376830ed-f0d3-40e7-8504-639e06eeb14b (Autodesk Fusion 360 design; units mm, degrees)
Autodesk Fusion 360 part; units mm, degrees
note: some values were not read from the file. Set by a fixed rule: which sketch regions a step uses.
sketch "Sketch1" plane through (0, 0, 0) normal (0, 1, 0) x (1, 0, 0)
  circle A0 centre (0, 0) radius 8.4709
  circle A1 centre (0, 0) radius 9.525
  circle A2 centre (0, 0) radius 7.412
  circle A3 centre (0, 0) radius 7.96
  arc A4 (9.5006, -0.6814) -> (-8.7304, -3.8087) centre (0, 0) ccw
  circle A5 centre (0, 0) radius 2.3813
  line L0 (0, 0) -> (9.525, 0) construction
  line L1 (0, 0) -> (-0.6938, -7.9298)
  line L2 (0, 0) -> (-1.3822, -7.8391)
  line L3 (0, 0) -> (-2.0602, -7.6888)
  line L4 (0, 0) -> (-2.7225, -7.48)
  line L5 (0, 0) -> (-3.3641, -7.2142)
  line L6 (0, 0) -> (-3.98, -6.8936)
  line L7 (0, 0) -> (-4.5657, -6.5205)
  line L8 (-0.6938, -7.9298) -> (-0.0018, -7.9903) construction
  line L9 (-1.3822, -7.8391) -> (-0.0141, -8.0804) construction
  line L10 (-2.0602, -7.6888) -> (-0.0473, -8.2282) construction
  line L11 (-2.7225, -7.48) -> (-0.1115, -8.4303) construction
  line L12 (-3.3641, -7.2142) -> (-0.2162, -8.6821) construction
  line L13 (-3.98, -6.8936) -> (-0.3705, -8.9775) construction
  line L14 (-4.5657, -6.5205) -> (-0.5826, -9.3095) construction
  line L15 (0, 0) -> (-5.1166, -6.0977)
  line L16 (-5.1166, -6.0977) -> (-0.8596, -9.6698) construction
  line L17 (0, 0) -> (-5.6286, -5.6286)
  line L18 (-5.6286, -5.6286) -> (-1.2079, -10.0493) construction
  spline S0 degree 5 poles (-1.2079, -10.0493) (-1.1965, -10.0361) (-1.1735, -10.01) (-1.139, -9.9713) (-1.0926, -9.9208) (-1.0346, -9.8592) (-0.9772, -9.7985) (-0.9208, -9.7382) (-0.8662, -9.678) (-0.8137, -9.6174) (-0.7634, -9.5563) (-0.7154, -9.4949) (-0.6695, -9.4332) (-0.6254, -9.3717) (-0.5829, -9.3104) (-0.5419, -9.2498) (-0.5022, -9.1898) (-0.4639, -9.1306) (-0.4271, -9.072) (-0.3918, -9.0141) (-0.3582, -8.9569) (-0.3264, -8.9002) (-0.2962, -8.8442) (-0.2677, -8.789) (-0.2409, -8.7347) (-0.2156, -8.6813) (-0.1919, -8.629) (-0.1697, -8.5779) (-0.1489, -8.5281) (-0.1297, -8.4795) (-0.112, -8.4323) (-0.0958, -8.3866) (-0.081, -8.3424) (-0.0676, -8.2999) (-0.0557, -8.2592) (-0.045, -8.2203) (-0.0356, -8.1835) (-0.0275, -8.1488) (-0.0206, -8.1164) (-0.015, -8.0864) (-0.0104, -8.059) (-0.0068, -8.0343) (-0.0041, -8.0127) (-0.0021, -7.9944) (-0.0007, -7.9796) (0.0002, -7.9687) (0.0004, -7.9631) (0.0003, -7.9609) (0.0001, -7.9602) (0, -7.96) knots 0 0 0 0 0 0 0.022222 0.044444 0.066667 0.088889 0.111111 0.133333 0.155556 0.177778 0.2 0.222222 0.244444 0.266667 0.288889 0.311111 0.333333 0.355556 0.377778 0.4 0.422222 0.444444 0.466667 0.488889 0.511111 0.533333 0.555556 0.577778 0.6 0.622222 0.644444 0.666667 0.688889 0.711111 0.733333 0.755556 0.777778 0.8 0.822222 0.844444 0.866667 0.888889 0.911111 0.933333 0.955556 0.977778 1 1 1 1 1 1
  line L19 (-1.3092, -10.166) -> (-1.1066, -9.9326)
  line L20 (0.0095, -7.9702) -> (-0.0095, -7.9499)
  line L21 (-0.1263, -8.47) -> (0, 0)
  line L22 (0, 0) -> (-0.6891, -6.0674) construction
  line L23 (0, -7.96) -> (0, 0) construction
  spline S1 degree 5 poles (0, -7.96) (0, -7.9287) (0, -7.8696) (0, -7.7913) (0, -7.7043) (0, -7.6106) (0, -7.5366) (0, -7.4767) (0, -7.434) (0, -7.412) knots 0 0 0 0 0 0 0.2 0.4 0.6 0.8 1 1 1 1 1 1
  spline S2 degree 5 poles (-1.785, -7.7573) (-1.7779, -7.7268) (-1.7647, -7.6691) (-1.7471, -7.5928) (-1.7276, -7.5081) (-1.7066, -7.4168) (-1.69, -7.3446) (-1.6766, -7.2863) (-1.667, -7.2447) (-1.6621, -7.2233) knots 0 0 0 0 0 0 0.2 0.4 0.6 0.8 1 1 1 1 1 1
  line L24 (0, -8.0339) -> (0, -7.8862)
  line L25 (0, -7.4639) -> (0, -7.3602)
  line L26 (-1.8015, -7.8293) -> (-1.7684, -7.6854)
  line L27 (-1.6737, -7.2738) -> (-1.6505, -7.1728)
  spline S3 degree 5 poles (-1.0763, -10.0642) (-1.0845, -10.0488) (-1.101, -10.0182) (-1.126, -9.9728) (-1.1599, -9.9132) (-1.2025, -9.8401) (-1.2449, -9.7681) (-1.2863, -9.6967) (-1.3261, -9.6258) (-1.3637, -9.5549) (-1.399, -9.4841) (-1.432, -9.4135) (-1.4629, -9.3431) (-1.492, -9.2732) (-1.5197, -9.2041) (-1.5461, -9.1358) (-1.5713, -9.0684) (-1.5953, -9.0021) (-1.6181, -8.9368) (-1.6395, -8.8725) (-1.6594, -8.8091) (-1.6778, -8.7467) (-1.6946, -8.6854) (-1.71, -8.6252) (-1.7239, -8.5662) (-1.7366, -8.5086) (-1.748, -8.4523) (-1.7582, -8.3975) (-1.7672, -8.3443) (-1.7751, -8.2927) (-1.7818, -8.2427) (-1.7873, -8.1945) (-1.7918, -8.1481) (-1.7953, -8.1037) (-1.7978, -8.0613) (-1.7995, -8.0211) (-1.8004, -7.9831) (-1.8005, -7.9475) (-1.7999, -7.9143) (-1.7987, -7.8838) (-1.797, -7.8561) (-1.795, -7.8312) (-1.7928, -7.8096) (-1.7906, -7.7913) (-1.7887, -7.7766) (-1.7871, -7.7657) (-1.786, -7.7602) (-1.7854, -7.758) (-1.7851, -7.7574) (-1.785, -7.7573) knots 0 0 0 0 0 0 0.022222 0.044444 0.066667 0.088889 0.111111 0.133333 0.155556 0.177778 0.2 0.222222 0.244444 0.266667 0.288889 0.311111 0.333333 0.355556 0.377778 0.4 0.422222 0.444444 0.466667 0.488889 0.511111 0.533333 0.555556 0.577778 0.6 0.622222 0.644444 0.666667 0.688889 0.711111 0.733333 0.755556 0.777778 0.8 0.822222 0.844444 0.866667 0.888889 0.911111 0.933333 0.955556 0.977778 1 1 1 1 1 1
  line L28 (-1.0038, -10.2006) -> (-1.1489, -9.9278)
  line L29 (-1.7965, -7.7651) -> (-1.7735, -7.7496)
  point P0 (-0.1263, -8.47)
  point P1 (0, -7.412)
  point P2 (-1.3307, -9.6163)
  point P3 (-1.5199, -9.2031)
  point P4 (-1.652, -8.832)
  point P5 (-1.7361, -8.5095)
  point P6 (-1.7818, -8.2406)
  point P7 (-1.799, -8.0292)
  point P8 (-1.7982, -7.8777)
  point P9 (-1.79, -7.7872)
  point P10 (-1.6621, -7.2233)
  dimension "d2" = 19.05
  dimension "id" = 14.8241
  dimension "BaseDiameter" = 15.9201
  dimension "d1" = 4.7625
  dimension "d34" = 5
  dimension "d35" = 5
  dimension "d36" = 5
  dimension "d37" = 5
  dimension "d38" = 5
  dimension "d39" = 5
  dimension "d41" = 0.6946
  dimension "d42" = 1.3893
  dimension "d43" = 2.0839
  dimension "d44" = 2.7786
  dimension "d45" = 3.4732
  dimension "d46" = 4.1679
  dimension "d47" = 4.8625
  dimension "d48" = 5
  dimension "d49" = 5.5572
  dimension "d50" = 5
  dimension "d51" = 6.2518
  dimension "d55" = 5.625
  dimension "d60" = 5
  constraint coincident A0.centre A1.centre
  constraint concentric A0 A2
  constraint coincident A1 A4.end
  constraint horizontal L0
  constraint coincident A4 L0.end
  constraint coincident A3 S0.end
  constraint coincident A3 L1.end
  constraint coincident A3 L2.end
  constraint coincident A3 L3.end
  constraint coincident A3 L4.end
  constraint coincident A3 L5.end
  constraint coincident A3 L6.end
  constraint coincident A3 L7.end
  constraint vertical A0.centre S0.end
  constraint tangent A3 L8
  constraint tangent A3 L9
  constraint tangent A3 L10
  constraint tangent A3 L11
  constraint tangent A3 L12
  constraint tangent A3 L13
  constraint tangent A3 L14
  constraint coincident A3 L15.end
  constraint tangent A3 L16
  constraint coincident A3 L17.end
  constraint tangent A3 L18
  constraint midpoint L18.end L19
  constraint midpoint S0.end L20
  constraint coincident A0 P0
  constraint coincident S0 P0
  constraint coincident P0 L21.start
  constraint coincident L23 P1
  constraint coincident A2 P1
  constraint coincident P1 S1.end
  constraint midpoint S0.end L24
  constraint midpoint P1 L25
  constraint symmetric S0.end L22 S2.start
  constraint symmetric L8.end L22 P9
  constraint symmetric L9.end L22 P8
  constraint symmetric L10.end L22 P7
  constraint symmetric L11.end L22 P6
  constraint symmetric L12.end L22 P5
  constraint symmetric L13.end L22 P4
  constraint symmetric L14.end L22 P3
  constraint symmetric L16.end L22 P2
  constraint symmetric L18.end L22 S3.start
  constraint symmetric L19.start L22 L28.start
  constraint symmetric L19.end L22 L28.end
  constraint symmetric L20.start L22 L29.start
  constraint symmetric L20.end L22 L29.end
  constraint symmetric L22 P1 P10
  constraint symmetric L22 L24.start L26.start
  constraint symmetric L22 L24.end L26.end
  constraint symmetric L22 L25.start L27.start
  constraint symmetric L22 L25.end L27.end
  constraint vertical L24
  constraint vertical L25
  measures "d2" diameter of A1
  measures "id" diameter of A2
  measures "BaseDiameter" diameter of A3
  measures "d1" diameter of A5
  measures "d34" angle of L1 L2
  measures "d35" angle of L2 L3
  measures "d36" angle of L3 L4
  measures "d37" angle of L4 L5
  measures "d38" angle of L5 L6
  measures "d39" angle of L6 L7
  measures "d41" distance of L1.end L8.end
  measures "d42" distance of L2.end L9.end
  measures "d43" distance of L3.end L10.end
  measures "d44" distance of L4.end L11.end
  measures "d45" distance of L5.end L12.end
  measures "d46" distance of L6.end L13.end
  measures "d47" distance of L7.end L14.end
  measures "d48" angle of L7 L15
  measures "d49" distance of L15.end L16.end
  measures "d50" angle of L15 L17
  measures "d51" distance of L17.end L18.end
  measures "d55" angle of L21 L22
  measures "d60" angle of L1 L23
extrude "Extrude1" add sketch "Sketch1" along normal blind 304.8 contours A0 A1 S0 S3 | A3 S0 L21 | A0 A3 L21 S3 | A2 A3 L21 S1 L24 L25 | A2 A3 L1 L21 | A2 A3 L2 S2 L26 L27 | A2 A3 L1 L2 makes body 1
pattern_circular "C-Pattern2" count 12 over 360 about axis through (0, 1.75, 0) along (0, 1, 0) of bodies 1 makes body 2 at (3.0432, 203.2, 6.7585) makes body 3 at (6.0147, 203.2, 4.3315) makes body 4 at (7.3746, 203.2, 0.7438) makes body 5 at (6.8328, 203.2, -2.8724) makes body 6 at (4.3315, 203.2, -6.0147) makes body 7 at (0.7438, 203.2, -7.3746) makes body 8 at (-3.0432, 203.2, -6.7585) makes body 9 at (-6.0147, 203.2, -4.3315) makes body 10 at (-7.3746, 203.2, -0.7438) makes body 11 at (-6.7585, 203.2, 3.0432) makes body 12 at (-4.3315, 203.2, 6.0147)
extrude "Extrude2" add sketch "Sketch1" along normal blind 304.8 contours A2 A5 L17 L21 | A2 A5 L1 L21 | A2 A5 L1 L2 | A2 A5 L2 L3 | A2 A5 L3 L4 | A2 A5 L15 L17 | A2 A5 L4 L5 | A2 A5 L7 L15 | A2 A5 L5 L6 | A2 A5 L6 L7 bodies 1 2 3 4 5 6 7 8 9 10 11 12
ref_plane "WorkPlane1" through (6.2747, 152.4, -0.8261) normal (0.130526, 0, 0.991445) x (0.991445, 0, -0.130526)
fillet "Fillet1" [suppressed]
mirror "Mirror3" [suppressed]
pattern_circular "C-Pattern1" [suppressed]
equation "d = 0.667 in"
equation "OutsideDiameter = d2"
equation "PitchDiameter = d"
equation "id = PitchDiameter - 2 * ( PitchDiameter / TeethNumber )"
equation "BaseDiameter = PitchDiameter * cos(20 deg)"
equation "Length = 12 in"
equation "t = 16"
equation "ShaftDiameter = d1"
equation "TeethNumber = t"
equation "Pitch = 32"
equation "d30 = ( 1.25 * ( PitchDiameter / TeethNumber ) ) - ( PitchDiameter / TeethNumber )"
equation "Basecircum = PI * PitchDiameter * cos(20 deg)"
equation "d41 = Basecircum * 5 / 360"
equation "d42 = Basecircum * 10 / 360"
equation "d43 = Basecircum * 15 / 360"
equation "d44 = Basecircum * 20 / 360"
equation "d45 = Basecircum * 25 / 360"
equation "d46 = Basecircum * 30 / 360"
equation "d47 = Basecircum * 35 / 360"
equation "d49 = Basecircum * 40 / 360"
equation "d51 = Basecircum * 45 / 360"
equation "d55 = ( 360 / ( 4 * TeethNumber ) ) * 1 deg"
